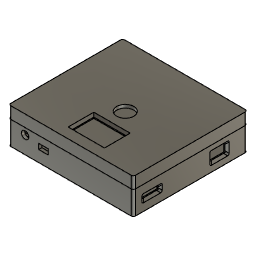
case v19 (Autodesk Fusion 360 design; units mm, degrees)
Autodesk Fusion 360 part; units mm, degrees
sketch "bottomsides" plane through (0, 0, 0) normal (0, 0, 1) x (1, 0, 0)
  line L0 (55.3, -50.3) -> (-55.3, -50.3)
  line L1 (-55.3, -50.3) -> (-55.3, 50.3)
  line L2 (-55.3, 50.3) -> (55.3, 50.3)
  line L3 (55.3, 50.3) -> (55.3, -50.3)
  line L4 (55.3, -50.3) -> (-55.3, 50.3) construction
  line L5 (-55.3, -50.3) -> (55.3, 50.3) construction
  line L6 (58.3, -53.3) -> (-58.3, -53.3)
  line L7 (-58.3, -53.3) -> (-58.3, 53.3)
  line L8 (-58.3, 53.3) -> (58.3, 53.3)
  line L9 (58.3, 53.3) -> (58.3, -53.3)
  dimension "case_width" = 110.6
  dimension "case_height" = 100.6
  dimension "d3" = -3
  constraint horizontal L0
  constraint perpendicular L0 L1
  constraint parallel L0 L2
  constraint parallel L1 L3
  constraint coincident L4 origin
  constraint coincident L5 origin
  measures "case_width" distance of L1.end L2.end
  measures "case_height" distance of L0.end L1.end
extrude "Extrude1" add sketch "bottomsides" along normal blind 22 makes body 1
extrude "Extrude2" add sketch "bottomsides" along normal blind 3 contours L0 L1 L2 L3 bodies 1
sketch "corners" plane through (0, 0, 3) normal (0, 0, 1) x (-1, 0, 0)
  line L0 (-55.3, -50.3) -> (55.3, -50.3)
  line L1 (55.3, -50.3) -> (55.3, 50.3)
  line L2 (55.3, 50.3) -> (-55.3, 50.3)
  line L3 (-55.3, 50.3) -> (-55.3, -50.3)
  line L4 (55.3, -50.3) -> (48.3, -50.3)
  line L5 (48.3, -50.3) -> (48.3, -43.3)
  line L6 (48.3, -43.3) -> (55.3, -43.3)
  line L7 (55.3, -43.3) -> (55.3, -50.3)
  line L8 (55.3, 50.3) -> (48.3, 50.3)
  line L9 (48.3, 50.3) -> (48.3, 43.3)
  line L10 (48.3, 43.3) -> (55.3, 43.3)
  line L11 (55.3, 43.3) -> (55.3, 50.3)
  line L12 (-55.3, 50.3) -> (-48.3, 50.3)
  line L13 (-48.3, 50.3) -> (-48.3, 43.3)
  line L14 (-48.3, 43.3) -> (-55.3, 43.3)
  line L15 (-55.3, 43.3) -> (-55.3, 50.3)
  line L16 (-55.3, -50.3) -> (-48.3, -50.3)
  line L17 (-48.3, -50.3) -> (-48.3, -43.3)
  line L18 (-48.3, -43.3) -> (-55.3, -43.3)
  line L19 (-55.3, -43.3) -> (-55.3, -50.3)
  dimension "d8" = 7
  dimension "d9" = 7
  dimension "d10" = 7
  dimension "d11" = 7
  dimension "d12" = 7
  dimension "d13" = 7
  dimension "d14" = 7
  dimension "d15" = 7
  constraint horizontal L4
  constraint vertical L5
  constraint horizontal L6
  constraint vertical L7
  constraint coincident L0.end L1.start
  constraint horizontal L8
  constraint vertical L9
  constraint horizontal L10
  constraint vertical L11
  constraint coincident L1.end L2.start
  constraint horizontal L12
  constraint vertical L13
  constraint horizontal L14
  constraint vertical L15
  constraint coincident L2.end L3.start
  constraint horizontal L16
  constraint vertical L17
  constraint horizontal L18
  constraint vertical L19
  constraint coincident L0.start L3.end
  measures "d8" distance of L0.end L4.end
  measures "d9" distance of L0.end L6.end
  measures "d10" distance of L1.end L8.end
  measures "d11" distance of L1.end L10.end
  measures "d12" distance of L2.end L12.end
  measures "d13" distance of L2.end L14.end
  measures "d14" distance of L0.start L16.end
  measures "d15" distance of L0.start L18.end
extrude "Extrude3" add sketch "corners" along normal blind 5 contours L0 L3 L16 L17 L18 L19 | L0 L1 L4 L5 L6 L7 | L2 L3 L12 L13 L14 L15 | L1 L2 L8 L9 L10 L11 bodies 1
fillet "Fillet1" radius 2 4 edges at (58.3, -53.3, 11) (58.3, 53.3, 11) (-58.3, -53.3, 11) (-58.3, 53.3, 11) on bodies 1
sketch "hole and switch" plane through (0, -53.3, 0) normal (0, -1, 0) x (1, 0, 0)
  line L0 (-56.3, 22) -> (-56.3, 0)
  line L1 (-56.3, 0) -> (56.3, 0)
  line L2 (56.3, 0) -> (56.3, 22)
  line L3 (56.3, 22) -> (-56.3, 22)
  circle A0 centre (-42.9, 16) radius 3.5
  line L4 (58.3, 0) -> (-58.3, 0)
  line L5 (-30.3, 15.6) -> (-21.3, 15.6)
  line L6 (-21.3, 15.6) -> (-21.3, 10.6)
  line L7 (-21.3, 10.6) -> (-30.3, 10.6)
  line L8 (-30.3, 10.6) -> (-30.3, 15.6)
  dimension "d20" = 7
  dimension "d21" = 13.4
  dimension "d22" = 16
  dimension "d23" = 9
  dimension "d24" = 5
  dimension "d25" = 10.6
  dimension "d26" = 26
  constraint horizontal L5
  constraint vertical L6
  constraint horizontal L7
  constraint vertical L8
  measures "d20" diameter of A0
  measures "d21" distance of L0 A0.centre
  measures "d22" distance of A0.centre L4
  measures "d23" distance of L5.start L5.end
  measures "d24" distance of L5.start L7.end
  measures "d25" distance of L4 L7
  measures "d26" distance of L0 L8
extrude "Extrude4" cut sketch "hole and switch" against normal up to surface (3 mm away) contours A0 | L5 L6 L7 L8 bodies 1
sketch "SD Slot USB C" plane through (58.3, 0, 0) normal (1, 0, 0) x (0, 1, 0)
  line L0 (51.3, 0) -> (51.3, 22)
  line L1 (51.3, 22) -> (-51.3, 22)
  line L2 (-51.3, 22) -> (-51.3, 0)
  line L3 (-51.3, 0) -> (51.3, 0)
  line L4 (-43.3, 12.4) -> (-28.3, 12.4)
  line L5 (-28.3, 12.4) -> (-28.3, 9)
  line L6 (-28.3, 9) -> (-43.3, 9)
  line L7 (-43.3, 9) -> (-43.3, 12.4)
  line L8 (20.3, 15.6) -> (34.3, 15.6)
  line L9 (34.3, 15.6) -> (34.3, 7.6)
  line L10 (34.3, 7.6) -> (20.3, 7.6)
  line L11 (20.3, 7.6) -> (20.3, 15.6)
  dimension "d29" = 15
  dimension "d30" = 3.4
  dimension "d31" = 9
  dimension "d32" = 8
  dimension "d33" = 8
  dimension "d34" = 14
  dimension "d35" = 7.6
  dimension "d36" = 17
  constraint horizontal L4
  constraint vertical L5
  constraint horizontal L6
  constraint vertical L7
  constraint horizontal L8
  constraint vertical L9
  constraint horizontal L10
  constraint vertical L11
  measures "d29" distance of L4.start L4.end
  measures "d30" distance of L4.start L6.end
  measures "d31" distance of L3 L6
  measures "d32" distance of L2 L7
  measures "d33" distance of L8.start L10.end
  measures "d34" distance of L9 L11
  measures "d35" distance of L3 L10
  measures "d36" distance of L0 L9
extrude "Extrude5" cut sketch "SD Slot USB C" against normal up to surface (3 mm away) contours L4 L5 L6 L7 | L8 L9 L10 L11 bodies 1
chamfer "Chamfer1" distance 2 angle 45 4 edges at (58.3, -35.8, 12.4) (58.3, -43.3, 10.7) (58.3, -35.8, 9) (58.3, -28.3, 10.7) on bodies 1
chamfer "Chamfer2" distance 2 angle 45 4 edges at (58.3, 20.3, 11.6) (58.3, 27.3, 15.6) (58.3, 34.3, 11.6) (58.3, 27.3, 7.6) on bodies 1
fillet "Fillet2" radius 2 4 edges at (57.3, 19.3, 16.6) (57.3, 35.3, 16.6) (57.3, 35.3, 6.6) (57.3, 19.3, 6.6) on bodies 1
fillet "Fillet3" radius 2 4 edges at (57.3, -44.3, 13.4) (57.3, -44.3, 8) (57.3, -27.3, 8) (57.3, -27.3, 13.4) on bodies 1
ref_plane "WorkPlane1" through (0, 0, 12.5) normal (1, 0, 0) x (0, 1, 0)
ref_plane "WorkPlane2" through (0, 0, 12.5) normal (0, -1, 0) x (1, 0, 0)
sketch "slots" plane through (0, 0, 0) normal (0, -1, 0) x (-1, 0, 0)
  line L0 (-55.3, -20) -> (-56.5, -18.8)
  line L1 (-56.5, -18.8) -> (-55.3, -17.6)
  line L2 (-55.3, -8) -> (-55.3, -22)
  line L3 (55.3, -17.6) -> (56.5, -18.8)
  line L4 (56.5, -18.8) -> (55.3, -20)
  line L5 (55.3, -8) -> (55.3, -22)
  line L6 (-56.3, -22) -> (56.3, -22)
  dimension "d50" = 2
  dimension "d51" = 90
  dimension "d52" = 1.2
  dimension "d57" = 90
  dimension "d58" = 2
  dimension "d59" = 1.2
  dimension "d114" = 45
  dimension "d115" = 45
  constraint coincident L0.start L2
  constraint coincident L1.end L2
  constraint coincident L4.end L5
  constraint coincident L3.start L5
  measures "d50" distance of L0.start L2.end
  measures "d51" angle of L0 L1
  measures "d52" distance of L0.end L2
  measures "d57" angle of L3 L4
  measures "d58" distance of L4.end L6
  measures "d59" distance of L3.end L5
  measures "d114" angle of L0 L2
  measures "d115" angle of L4 L5
extrude "Extrude6" cut sketch "slots" along normal mid plane 40 contours L0 L1 L2 bodies 1
extrude "Extrude7" cut sketch "slots" along normal mid plane 40 contours L3 L4 L5 bodies 1
copy_body "Body->Comp1" bodies 1 removing the originals makes body 2 in component "CaseBottom"
sketch "top" plane through (0, 0, 0) normal (0, 0, 1) x (1, 0, 0) in component "CaseTop"
  line L0 (0, 0) -> (110.6, 0)
  line L1 (110.6, 0) -> (110.6, -100.6)
  line L2 (110.6, -100.6) -> (0, -100.6)
  line L3 (0, -100.6) -> (0, 0)
  line L4 (-3, -103.6) -> (-3, 3)
  line L5 (-3, 3) -> (113.6, 3)
  line L6 (113.6, 3) -> (113.6, -103.6)
  line L7 (113.6, -103.6) -> (-3, -103.6)
  circle A0 centre (57, -46) radius 8
  line L8 (109.4, -99.4) -> (1.2, -99.4)
  line L9 (1.2, -99.4) -> (1.2, -1.2)
  line L10 (1.2, -1.2) -> (109.4, -1.2)
  line L11 (109.4, -1.2) -> (109.4, -99.4)
  dimension "d64" = 110.6
  dimension "d65" = 100.6
  dimension "d66" = -3
  dimension "d67" = 16
  dimension "d68" = 57
  dimension "d74" = 46
  dimension "d80" = 1.2
  constraint horizontal L0
  constraint vertical L1
  constraint horizontal L2
  constraint vertical L3
  constraint coincident L0.start L3.end
  measures "d64" distance of L0.start L0.end
  measures "d65" distance of L0 L2
  measures "d67" diameter of A0
  measures "d68" distance of L3 A0.centre
  measures "d74" distance of L0 A0.centre
extrude "Extrude1'" add sketch "top" against normal blind 3 separate body contours L0 L1 L2 L3 | L4 L5 L6 L7 | A0 | L8 L9 L10 L11 makes body 3 in component "CaseTop"
extrude "Extrude2'" cut sketch "top" against normal through all contours A0 bodies 3 in component "CaseTop"
extrude "Extrude3'" add sketch "top" along normal blind 8 contours L4 L5 L6 L7 bodies 3 in component "CaseTop"
sketch "bezel" plane through (0, 0, 0) normal (0, 0, 1) x (1, 0, 0) in component "CaseTop"
  line L0 (45, -8.6) -> (75, -8.6)
  line L1 (75, -8.6) -> (75, -28.6)
  line L2 (75, -28.6) -> (45, -28.6)
  line L3 (45, -28.6) -> (45, -8.6)
  line L4 (0, -100.6) -> (0, 0)
  line L5 (0, 0) -> (110.6, 0)
  dimension "d75" = 20
  dimension "d76" = 30
  dimension "d77" = 45
  dimension "d78" = 8.6
  constraint horizontal L0
  constraint vertical L1
  constraint horizontal L2
  constraint vertical L3
  measures "d75" distance of L0 L2
  measures "d76" distance of L1 L3
  measures "d77" distance of L3 L4
  measures "d78" distance of L0 L5
extrude "Extrude4'" cut sketch "bezel" against normal through all bodies 3 in component "CaseTop"
extrude "Extrude5'" add sketch "top" along normal blind 13 contours L0 L1 L2 L3 bodies 3 in component "CaseTop"
fillet "Fillet1'" radius 2 4 edges at (-3, -103.6, 2.5) (113.6, -103.6, 2.5) (113.6, 3, 2.5) (-3, 3, 2.5) on bodies 3 in component "CaseTop"
sketch "antenna cutout" plane through (0, -1.2, 0) normal (0, -1, 0) x (1, 0, 0)
  line L0 (1.2, 0) -> (109.4, 0)
  line L1 (109.4, 0) -> (109.4, 13)
  line L2 (109.4, 13) -> (1.2, 13)
  line L3 (1.2, 13) -> (1.2, 0)
  line L4 (7.7, 13) -> (7.7, 11.8)
  arc A0 (7.7, 11.8) -> (16.7, 11.8) centre (12.2, 11.8) ccw
  line L5 (16.7, 11.8) -> (16.7, 13)
  dimension "d96" = 1.2
  dimension "d97" = 11
  dimension "d98" = 9
  constraint coincident L2 L4.start
  constraint perpendicular L2 L4
  constraint tangent L4 A0
  constraint coincident L2 L5.end
  constraint tangent A0 L5
  constraint perpendicular L2 L5
  measures "d96" distance of L2 A0.centre
  measures "d97" distance of L3 A0.centre
  measures "d98" distance of L4 L5
move_body "Move1" bodies 3 to x (-1, 0, 0) y (0, 1, 0) z (0, 0, -1) at (227.2, 0, 16) in component "CaseTop"
move_body "Move2" bodies 3 to x (-1, 0, 0) y (0, -1, 0) z (0, 0, 1) at (231.2, 2, 0) in component "CaseTop"
move_body "Move3" bodies 3 to x (1, 0, 0) y (0, 1, 0) z (0, 0, 1) at (-60, -50, 0) in component "CaseTop"
move_body "Move4" bodies 3 to x (1, 0, 0) y (0, 1, 0) z (0, 0, 1) at (0, 0, 15) in component "CaseTop"
ref_plane "WorkPlane1" through (-0.7, 2.3, 28.5) normal (0, 1, 0) x (-1, 0, 0) in component "CaseTop"
sketch "antenna switch clearance" plane through (0, -46.8, 0) normal (0, 1, 0) x (-1, 0, 0) in component "CaseTop"
  line L0 (54.8, 31) -> (-53.4, 31)
  line L1 (-53.4, 31) -> (-53.4, 18)
  line L2 (-53.4, 18) -> (54.8, 18)
  line L3 (54.8, 18) -> (54.8, 31)
  line L4 (50.0343, 18) -> (22.0343, 18)
  line L5 (22.0343, 18) -> (22.0343, 22)
  line L6 (22.0343, 22) -> (50.0343, 22)
  line L7 (50.0343, 22) -> (50.0343, 18)
  dimension "d131" = 28
  dimension "d132" = 4
  constraint horizontal L4
  constraint vertical L5
  constraint horizontal L6
  constraint vertical L7
  constraint coincident L2 L4.start
  measures "d131" distance of L4.start L4.end
  measures "d132" distance of L4.start L6.end
extrude "Extrude16" cut sketch "antenna switch clearance" against normal up to surface (1.2 mm away) contours L2 L4 L5 L6 L7 bodies 3 in component "CaseTop"
fillet "Fillet5" radius 1 2 edges at (-22.0343, -47.4, 18) (-50.0343, -47.4, 18) on bodies 3 in component "CaseTop"
fillet "Fillet6" radius 1 2 edges at (-22.0343, -47.4, 22) (-50.0343, -47.4, 22) on bodies 3 in component "CaseTop"
extrude "Extrude17" cut 1 faces at (29.3886, -48, 19.6667) along direction (0, 1, 0) blind 0.1 on bodies 3 bodies 3 in component "CaseTop"
extrude "Extrude18" cut 1 faces at (17.7333, 52.6, 21.3333) along direction (0, -1, 0) blind 0.1 on bodies 3 bodies 3 in component "CaseTop"
extrude "Extrude19" cut 1 faces at (54.6, -14.4333, 19.6667) along direction (-1, 0, 0) blind 0.1 on bodies 3 bodies 3 in component "CaseTop"
extrude "Extrude20" cut 1 faces at (-56, 19.0333, 19.6667) along direction (1, 0, 0) blind 0.1 on bodies 3 bodies 3 in component "CaseTop"
fillet "Fillet7" radius 0.6 4 edges at (-55.9, -47.9, 20.5) (54.5, -47.9, 20.5) (-55.9, 52.5, 20.5) (54.5, 52.5, 20.5) on bodies 3 in component "CaseTop"
sketch "lips" plane through (0, 2.3, 0) normal (0, 1, 0) x (1, 0, 0) in component "CaseTop"
  line L0 (54.5, -21) -> (55.5, -20)
  line L1 (55.5, -20) -> (54.5, -19)
  line L2 (54.5, -18) -> (54.5, -23)
  line L3 (-55.9, -21) -> (-56.9, -20)
  line L4 (-56.9, -20) -> (-55.9, -19)
  line L5 (-55.9, -23) -> (-55.9, -18)
  dimension "d150" = 2
  dimension "d151" = 2
  dimension "d152" = 45
  dimension "d153" = 2
  dimension "d154" = 2
  dimension "d155" = 45
  constraint perpendicular L0 L1
  constraint coincident L0.start L2
  constraint coincident L1.end L2
  constraint perpendicular L3 L4
  constraint coincident L3.start L5
  constraint coincident L4.end L5
  measures "d150" distance of L0.start L1.end
  measures "d151" distance of L0.start L2.end
  measures "d152" angle of L3 L5
  measures "d153" distance of L3.start L5.start
  measures "d154" distance of L3.start L4.end
  measures "d155" angle of L0 L2
extrude "Extrude21" add sketch "lips" along normal mid plane 32 bodies 3 in component "CaseTop"
chamfer "Chamfer3" distance 2 angle 45 4 edges at (4, -39.4, 34) (19, -29.4, 34) (4, -19.4, 34) (-11, -29.4, 34) on bodies 3 in component "CaseTop"
component "CaseTop" placed x (1, 0, 0) y (0, 1, 0) z (0, 0, 1) at (0.7, -2.3, -1)
component "CaseBottom" placed x (1, 0, 0) y (0, 1, 0) z (0, 0, 1) at (0, 0, 0)
equation "case_width = 112 mm - 1.4 mm"
equation "case_height = 102 mm - 1.4 mm"
equation "d8 = corner_size"
equation "d9 = corner_size"
equation "d10 = corner_size"
equation "d11 = corner_size"
equation "d12 = corner_size"
equation "d13 = corner_size"
equation "d14 = corner_size"
equation "d15 = corner_size"
equation "d25 = 11 mm - 0.4 mm"
equation "d30 = 4 mm - 0.6 mm"
equation "corner_size = 7 mm"
equation "slot_length = 20 mm"
equation "slot_offset = 2 mm"
equation "slot_width = 1.6 mm"
equation "slot_depth = 1.2 mm"
equation "d50 = slot_offset"
equation "d52 = slot_depth"
equation "d53 = slot_length"
equation "d58 = slot_offset"
equation "d59 = slot_depth"
equation "d60 = slot_length"
equation "d64 = case_width"
equation "d65 = case_height"
equation "d78 = 9.6 mm - 1 mm"
equation "top_clearance = -0.1 mm"
equation "d150 = slot_width + 0.4 mm"
equation "d151 = slot_offset"
equation "d153 = slot_offset"
equation "d154 = slot_width + 0.4 mm"
equation "d156 = slot_length * 0.8"
named bodies: "FoxCase", "FoxCaseBottom", "FoxCaseTop"
